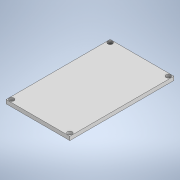
# Autodesk Inventor part: PCB_BOARD_NO_DREMEL_HOLES
Saved by Autodesk Inventor 2021 (Build 250183000, 183)
## iProperties
Created: 2021-04-21
Part Number: PCB_BOARD_NO_DREMEL_HOLES
Material: Generic
Document SubType Name: Modeling
Designer: Patrick
Density: 1 g/cm^3
Appearance: Default
Author: Patrick
Autodesk Inventor part; units mm, degrees
ref_plane "YZ Plane" through (0, 0, 0) normal (1, 0, 0) x (0, 1, 0)
ref_plane "XZ Plane" through (0, 0, 0) normal (0, 1, 0) x (-1, 0, 0)
ref_plane "XY Plane" through (0, 0, 0) normal (0, 0, 1) x (1, 0, 0)
sketch "Sketch1" plane through (0, 0, 0) normal (0, 1, 0) x (-1, 0, 0)
  line L0 (0, 0) -> (43.18, 0)
  line L1 (43.18, 0) -> (43.18, -70.49)
  line L2 (43.18, -70.49) -> (0, -70.49)
  line L3 (0, -70.49) -> (0, 0)
  circle A0 centre (41.27, -1.91) radius 1.5875
  circle A1 centre (41.27, -68.58) radius 1.5875
  circle A2 centre (1.91, -1.91) radius 1.5875
  circle A3 centre (1.91, -68.58) radius 1.5875
  dimension "d0" = 70.49
  dimension "d1" = 43.18
  dimension "d3" = 3.175
  dimension "d4" = 3.175
  dimension "d6" = 1.91
  dimension "d7" = 1.91
  dimension "d8" = 1.91
  dimension "d9" = 3.175
  dimension "d10" = 3.175
  dimension "d11" = 1.91
  dimension "d12" = 1.91
  dimension "d13" = 1.91
  dimension "d14" = 1.91
  dimension "d15" = 1.91
  constraints: 8 end point, 4 centre point, 2 parallel, 1 horizontal, 1 perpendicular
  measures "d0" distance of L2.end L0.start
  measures "d1" distance between parallel lines of L3 L1
  measures "d3" diameter of A1
  measures "d4" diameter of A0
  measures "d6" distance from line of L1 A0.centre
  measures "d7" distance from line of L2 A1.centre
  measures "d8" distance from line of A0.centre L0
  measures "d9" diameter of A2
  measures "d10" diameter of A3
  measures "d11" distance from line of L0 A2.centre
  measures "d12" distance from line of A2.centre L3
  measures "d13" distance from line of L2 A3.centre
  measures "d14" distance from line of L3 A3.centre
  measures "d15" distance from line of L1 A1.centre
extrude "Extrusion1" add sketch "Sketch1" along normal blind 2.54
body "Solid1"
